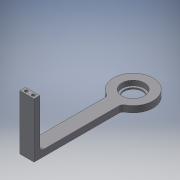
# Autodesk Inventor part: test_arm
Saved by Autodesk Inventor 2019.4 (Build 234330000, 330)
## iProperties
Created: 2019-08-15
Part Number: test_arm
Material: 일반
Document SubType Name: Modeling
Designer: cdi
Density: 1 g/cm^3
Appearance: 기본값
Author: cdi
Autodesk Inventor part; units mm, degrees
ref_plane "YZ Plane" through (0, 0, 0) normal (1, 0, 0) x (0, 1, 0)
ref_plane "XZ Plane" through (0, 0, 0) normal (0, 1, 0) x (-1, 0, 0)
ref_plane "XY Plane" through (0, 0, 0) normal (0, 0, 1) x (1, 0, 0)
sketch "스케치1" plane through (0, 0, 0) normal (0, 1, 0) x (-1, 0, 0)
  circle A0 centre (0, 0) radius 16.025
  circle A1 centre (0, 0) radius 28
  dimension "d0" = 32.05
  dimension "d1" = 56
  constraints: 2 centre point, 2 coincident
  measures "d0" diameter of A0
  measures "d1" diameter of A1
extrude "돌출1" add sketch "스케치1" along normal blind 9
sketch "스케치2" plane through (0, 0, 0) normal (0, -1, 0) x (1, 0, 0)
  circle A0 centre (0, 0) radius 13
  circle A1 centre (0, 0) radius 16.025 projected
  dimension "d4" = 26
  constraints: 1 centre point, 1 coincident
  measures "d4" diameter of A0
extrude "돌출2" add sketch "스케치2" against normal blind 2
sketch "스케치3" plane through (0, 0, 0) normal (0, -1, 0) x (1, 0, 0)
  circle A0 centre (0, 0) radius 28 projected
  line L0 (-10, 26.1534) -> (10, 26.1534)
  line L1 (10, 26.1534) -> (10, 150)
  line L2 (10, 150) -> (-10, 150)
  line L3 (-10, 150) -> (-10, 26.1534)
  dimension "d7" = 20
  dimension "d8" = 10
  dimension "d15" = 150
  constraints: 8 end point, 2 parallel, 2 point on circle, 1 horizontal, 1 perpendicular
  measures "d7" distance between parallel lines of L3 L1
  measures "d8" distance from line of point (0, 0) L1
  measures "d15" distance from line of point (0, 0) L2
extrude "돌출3" add sketch "스케치3" against normal up to surface (9 mm away) contours A0 L3 L2 L1
sketch "스케치4" plane through (0, 9, 0) normal (0, 1, 0) x (1, 0, 0)
  line L0 (10, -150) -> (-10, -150) projected
  line L1 (10, -150) -> (-10, -150)
  line L2 (-10, -150) -> (-10, -142)
  line L3 (-10, -142) -> (10, -142)
  line L4 (10, -142) -> (10, -150)
  point P0 (0, 0)
  dimension "d12" = 8
  constraints: 8 end point, 2 parallel, 1 horizontal, 1 perpendicular
  measures "d12" distance of L1.end L2.end
extrude "돌출4" add sketch "스케치4" along normal blind 69
fillet "모깎기1" radius 6 2 edges at (10, 4.5, 26.1534) (-10, 4.5, 26.1534)
sketch "스케치5" plane through (0, 78, 0) normal (0, 1, 0) x (1, 0, 0)
  circle A0 centre (-5, -146) radius 1.55 projected
  circle A1 centre (5, -146) radius 1.55 projected
  point P0 (0, 0)
hole "구멍1" at (-5, 78, 146) at (5, 78, 146) direction (0, -1, 0) diameter 3.88 depth 10 tip angle 118 countersink diameter 4.34 countersink angle 7
fillet "모깎기2" radius 6 1 edges at (0, 9, 142)
